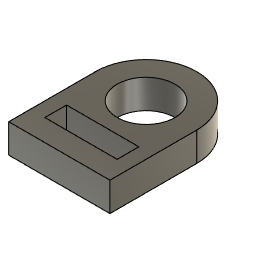
Exercise_01 (Autodesk Fusion 360 design; units mm, degrees)
Autodesk Fusion 360 part; units mm, degrees
sketch "Sketch1" plane through (0, 0, 0) normal (0, 0, 1) x (1, 0, 0)
  line L0 (70, 50) -> (70, -10)
  line L1 (70, -10) -> (0, -10)
  line L2 (0, -10) -> (0, 50)
  circle A0 centre (35, 50) radius 20
  arc A1 (70, 50) -> (0, 50) centre (35, 50) ccw
  line L3 (10, 5) -> (60, 5)
  line L4 (60, 5) -> (60, 20)
  line L5 (60, 20) -> (10, 20)
  line L6 (10, 20) -> (10, 5)
  dimension "d1" = 40
  constraint vertical L0
  constraint horizontal L1
  constraint vertical L2
  constraint concentric A0 A1
  constraint horizontal L3
  constraint vertical L4
  constraint horizontal L5
  constraint vertical L6
  measures "d1" diameter of A0
extrude "Extrude1" add sketch "Sketch1" along normal blind 20
